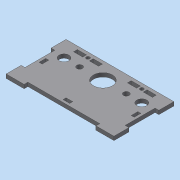
# Autodesk Inventor part: X-Anchor_Front-Inner
Saved by Autodesk Inventor 2016 SP1 (Build 200210100, 210)
## iProperties
Created: 2015-12-01
Part Number: X-Anchor_Front-Inner
Material: Generic
Document SubType Name: Modeling
Designer: Mohamed A.
Density: 1 g/cm^3
Appearance: Default
Author: Mohamed A.
Autodesk Inventor part; units mm, degrees
ref_plane "YZ Plane" through (0, 0, 0) normal (1, 0, 0) x (0, 1, 0)
ref_plane "XZ Plane" through (0, 0, 0) normal (0, 1, 0) x (-1, 0, 0)
ref_plane "XY Plane" through (0, 0, 0) normal (0, 0, 1) x (1, 0, 0)
sketch "Sketch1" plane through (0, 0, 0) normal (0, 0, 1) x (1, 0, 0)
  circle A0 centre (0, 5) radius 7.5
  line L0 (42.7333, 18.5) -> (-42.7333, 18.5)
  line L1 (-42.7333, -29) -> (42.7333, -29)
  circle A1 centre (18.5, 5) radius 2.25
  circle A2 centre (-18.5, 5) radius 2.25
  circle A3 centre (30.8333, 5) radius 3.9
  circle A4 centre (-30.8333, 5) radius 3.9
  line L2 (42.7333, 18.5) -> (42.7333, -29)
  line L3 (-42.7333, -29) -> (-42.7333, 18.5)
  circle A5 centre (0, 5) radius 13.5 construction
  line L4 (0, 41.7106) -> (0, -39.2634) construction
  dimension "d2" = 4.5
  dimension "d3" = 4.5
  dimension "d4" = 7.8
  dimension "d5" = 7.8
  dimension "d48" = 47.5
  dimension "d58" = 15
  dimension "d63" = 27
  dimension "d75" = 34
  dimension "d76" = 30.8333
  dimension "d77" = 85.4667
  dimension "d93" = 47.5
  constraints: 10 end point, 6 centre point, 3 vertical, 1 coincident, 1 perpendicular, 1 point on line, 6 other
  measures "d2" diameter of A1
  measures "d3" diameter of A2
  measures "d4" diameter of A3
  measures "d5" diameter of A4
  measures "d48" distance between parallel lines of L1 L0
  measures "d58" diameter of A0
  measures "d63" diameter of A5
  measures "d75" distance from line of A0.centre L1
  measures "d76" distance from line of A3.centre L4
  measures "d77" distance between parallel lines of L3 L2
  measures "d93" distance of L0.start L1.end
extrude "Extrusion1" add sketch "Sketch1" against normal blind 3
sketch "Sketch4" plane through (0, 0, 0) normal (0, 0, 1) x (1, 0, 0)
  line L0 (-42.7333, -29) -> (42.7333, -29) projected
  line L1 (42.7333, 18.5) -> (-42.7333, 18.5) projected
  line L2 (50.1623, -5.25) -> (-50.4474, -5.25) construction
  line L3 (42.7333, -29) -> (42.7333, 18.5) projected
  circle A0 centre (0, 5) radius 13.5 construction
  circle A1 centre (0, 5) radius 7.5 projected
  line L4 (42.7333, 6.625) -> (39.7333, 6.625)
  line L5 (39.7333, 6.625) -> (39.7333, -17.125)
  line L6 (39.7333, -17.125) -> (42.7333, -17.125)
  line L7 (42.7333, -17.125) -> (42.7333, 6.625)
  line L8 (0, 33.7344) -> (0, -36.9537) construction
  line L9 (-42.7333, 18.5) -> (-42.7333, -29) projected
  line L10 (-42.7333, 6.625) -> (-39.7333, 6.625)
  line L11 (-39.7333, 6.625) -> (-39.7333, -17.125)
  line L12 (-39.7333, -17.125) -> (-42.7333, -17.125)
  line L13 (-42.7333, -17.125) -> (-42.7333, 6.625)
  line L14 (42.7333, -29) -> (-42.7333, -29) projected
  line L15 (31.3, 16) -> (24.0167, 16) construction
  line L16 (11.4333, 16) -> (11.4333, 13) construction
  line L17 (11.4333, 13) -> (18.7167, 13) construction
  line L18 (31.3, 13) -> (31.3, 16) construction
  circle A2 centre (30.8333, 5) radius 3.9 projected
  line L19 (21.3667, 17.602) -> (21.3667, 7.8585) construction
  line L20 (18.7167, 16) -> (24.0167, 16) construction
  line L21 (24.0167, 16) -> (24.0167, 13) construction
  line L22 (24.0167, 13) -> (18.7167, 13) construction
  line L23 (18.7167, 13) -> (18.7167, 16) construction
  line L24 (18.7167, 16) -> (11.4333, 16) construction
  line L25 (24.0167, 13) -> (31.3, 13) construction
  circle A3 centre (21.3667, 14.5) radius 1.4
  line L26 (-31.3, 16) -> (-24.0167, 16) construction
  line L27 (-11.4333, 16) -> (-11.4333, 13) construction
  line L28 (-11.4333, 13) -> (-18.7167, 13) construction
  line L29 (-31.3, 13) -> (-31.3, 16) construction
  line L30 (-24.0167, 16) -> (-24.0167, 13) construction
  line L31 (-18.7167, 13) -> (-18.7167, 16) construction
  line L32 (-18.7167, 16) -> (-11.4333, 16) construction
  line L33 (-24.0167, 13) -> (-31.3, 13) construction
  circle A4 centre (-21.3667, 14.5) radius 1.4
  line L34 (42.7333, 18.5) -> (42.7333, -29) projected
  line L35 (-28.4889, -26) -> (28.4889, -26)
  line L36 (28.4889, -26) -> (28.4889, -29)
  line L37 (28.4889, -29) -> (-28.4889, -29)
  line L38 (-28.4889, -29) -> (-28.4889, -26)
  line L39 (35.3333, -2.6) -> (37.7333, -2.6)
  line L40 (37.7333, -2.6) -> (37.7333, -7.9)
  line L41 (37.7333, -7.9) -> (35.3333, -7.9)
  line L42 (35.3333, -7.9) -> (35.3333, -2.6)
  line L43 (-35.3333, -2.6) -> (-37.7333, -2.6)
  line L44 (-37.7333, -2.6) -> (-37.7333, -7.9)
  line L45 (-37.7333, -7.9) -> (-35.3333, -7.9)
  line L46 (-35.3333, -7.9) -> (-35.3333, -2.6)
  line L47 (2.65, -21.6) -> (-2.65, -21.6)
  line L48 (-2.65, -21.6) -> (-2.65, -24)
  line L49 (-2.65, -24) -> (2.65, -24)
  line L50 (2.65, -24) -> (2.65, -21.6)
  line L51 (-42.7333, -29) -> (-42.7333, 18.5) projected
  line L52 (-42.7333, -29) -> (-39.7333, -29)
  line L53 (-39.7333, -29) -> (-39.7333, -26)
  line L54 (-39.7333, -26) -> (-42.7333, -26)
  line L55 (-42.7333, -26) -> (-42.7333, -29)
  line L56 (42.7333, -29) -> (39.7333, -29)
  line L57 (39.7333, -29) -> (39.7333, -26)
  line L58 (39.7333, -26) -> (42.7333, -26)
  line L59 (42.7333, -26) -> (42.7333, -29)
  line L60 (11.4247, 13) -> (11.4247, 16)
  line L61 (11.4247, 16) -> (18.7077, 16)
  line L62 (18.7077, 16) -> (18.7077, 13)
  line L63 (18.7077, 13) -> (11.4247, 13)
  line L64 (31.2907, 16) -> (31.2907, 13)
  line L65 (31.2907, 13) -> (24.0077, 13)
  line L66 (24.0077, 13) -> (24.0077, 16)
  line L67 (24.0077, 16) -> (31.2907, 16)
  line L68 (-18.7073, 13) -> (-18.7073, 16)
  line L69 (-18.7073, 16) -> (-11.4243, 16)
  line L70 (-11.4243, 16) -> (-11.4243, 13)
  line L71 (-11.4243, 13) -> (-18.7073, 13)
  line L72 (-24.0073, 16) -> (-24.0073, 13)
  line L73 (-24.0073, 13) -> (-31.2903, 13)
  line L74 (-31.2903, 13) -> (-31.2903, 16)
  line L75 (-31.2903, 16) -> (-24.0073, 16)
  dimension "d61" = 47.5
  dimension "d62" = 27
  dimension "d81" = 3
  dimension "d82" = 11
  dimension "d83" = 19.8667
  dimension "d86" = 85.4667
  dimension "d88" = 5.3
  dimension "d89" = 2.8
  dimension "d97" = 23.75
  dimension "d98" = 3
  dimension "d99" = 3
  dimension "d100" = 56.9778
  dimension "d101" = 2.4
  dimension "d102" = 5.3
  dimension "d103" = 5
  dimension "d104" = 2.4
  dimension "d105" = 5.3
  dimension "d106" = 5
  dimension "d107" = 5.3
  dimension "d108" = 2.4
  dimension "d109" = 5
  constraints: 138 end point, 21 parallel, 20 horizontal, 13 symmetric about line, 10 perpendicular, 10 vertical, 6 collinear, 3 centre point, 3 point on line, 1 concentric, 25 other
  measures "d61" distance between parallel lines of L0 L1
  measures "d62" diameter of A0
  measures "d81" distance of L16.end L16.start
  measures "d82" distance from line of L15 A2.centre
  measures "d83" distance between parallel lines of L16 L18
  measures "d86" distance between parallel lines of L9 L3
  measures "d88" distance of L21.end L17.end
  measures "d89" diameter of A3
  measures "d97" distance between parallel lines of L6 L4
  measures "d98" distance between parallel lines of L3 L5
  measures "d99" distance between parallel lines of L0 L35
  measures "d100" distance between parallel lines of L38 L36
  measures "d101" distance of L40.end L41.end
  measures "d102" distance of L39.end L40.end
  measures "d103" distance between parallel lines of L3 L40
  measures "d104" distance of L45.end L44.end
  measures "d105" distance of L44.end L43.end
  measures "d106" distance between parallel lines of L13 L44
  measures "d107" distance of L49.end L48.end
  measures "d108" distance of L48.end L47.end
  measures "d109" distance between parallel lines of L37 L49
extrude "Extrusion2" cut sketch "Sketch4" against normal through all contours L38 L35 L36 L0 | L9 L10 L11 L12 | L3 L6 L5 L4 | A1 | A2 | A3 | A4 | L39 L40 L41 L42 | L46 L45 L44 L43 | L50 L49 L48 L47 | L60 L61 L62 L63 | L64 L65 L66 L67 | L68 L69 L70 L71 | L72 L73 L74 L75
equation "\"d48\" = d75 + 0.5 * d63"
body "Solid1"
